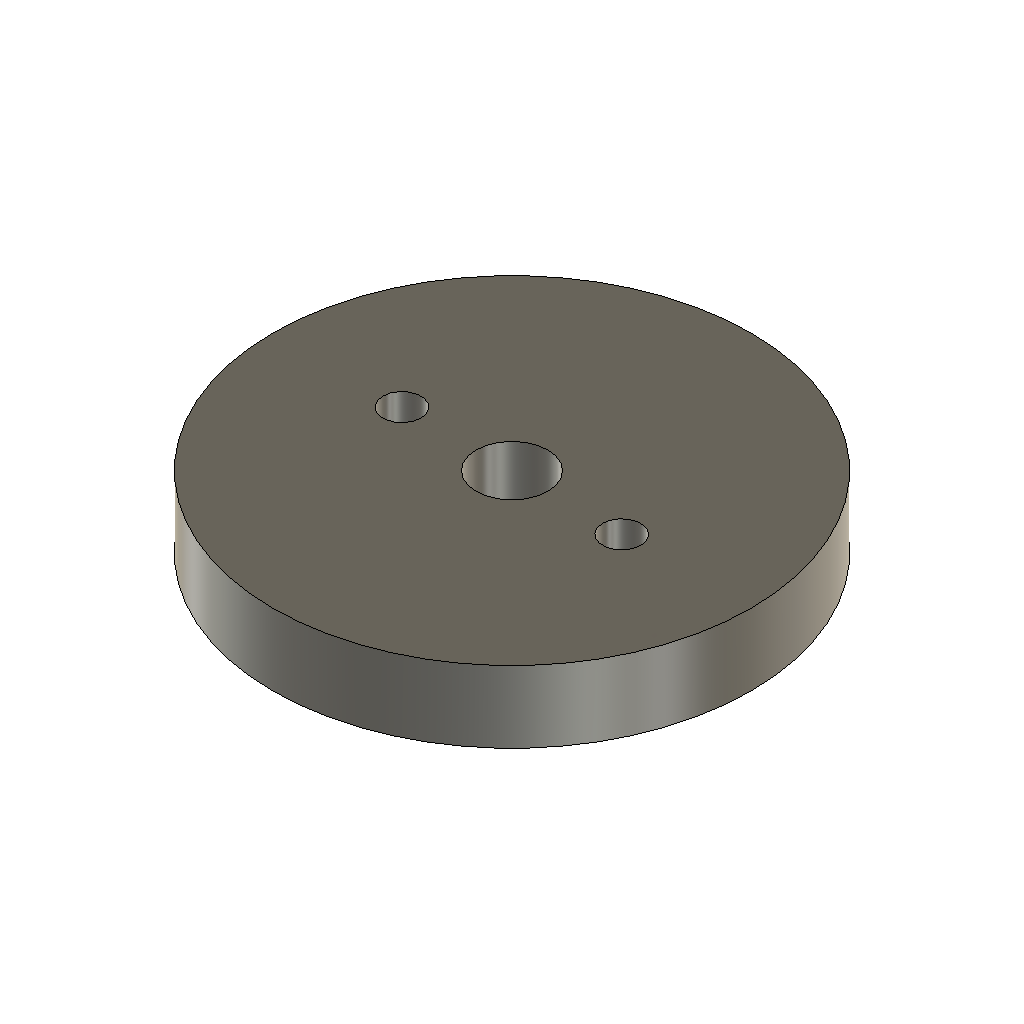
frontplate (Autodesk Fusion 360 design; units mm, degrees)
part number: 2026-09-10-22-39-12-020
Autodesk Fusion 360 part; units mm, degrees
sketch "Sketch1" plane through (0, 0, 0) normal (0, 0, 1) x (1, 0, 0)
  circle A0 centre (0, 0) radius 10
  dimension "d1" = 20
  constraint coincident A0.centre origin
  measures "d1" diameter of A0
extrude "Extrude1" add sketch "Sketch1" along normal blind 3
sketch "Sketch2" plane through (0, 0, 3) normal (0, 0, 1) x (-1, 0, 0)
  circle A0 centre (0, 0) radius 10
  circle A1 centre (0, 0) radius 1.5
  dimension "d4" = 3
  constraint coincident A0.centre A1.centre
  measures "d4" diameter of A1
extrude "Extrude2" cut sketch "Sketch2" against normal blind 12 contours A1
sketch "Sketch3" plane through (0, 0, 3) normal (0, 0, 1) x (-1, 0, 0)
  circle A0 centre (0, 0) radius 1.5
  circle A1 centre (0, 0) radius 10
  circle A2 centre (-4.6093, 0.0139) radius 0.8
  dimension "d7" = 1.6
  measures "d7" diameter of A2
sketch "Sketch4" plane through (0, 0, 3) normal (0, 0, 1) x (-1, 0, 0)
  circle A0 centre (4.6091, 0) radius 0.8
  dimension "d8" = 1.6
  measures "d8" diameter of A0
extrude "Extrude3" cut sketch "Sketch3" sketch "Sketch4" against normal blind 3 contours A2 of sketch 2
